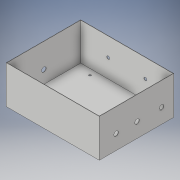
# Autodesk Inventor part: 563-AC-1404-5x4-Enclosure
Saved by Autodesk Inventor 2018 (Build 220112000, 112)
## iProperties
Created: 2018-04-30
Part Number: 563-AC-1404-5x4-Enclosure
Material: Generic
Document SubType Name: Modeling
Designer: bbramman
Density: 1 g/cm^3
Appearance: Default
Author: bbramman
Autodesk Inventor part; units mm, degrees
ref_plane "YZ Plane" through (0, 0, 0) normal (1, 0, 0) x (0, 1, 0)
ref_plane "XZ Plane" through (0, 0, 0) normal (0, 1, 0) x (-1, 0, 0)
ref_plane "XY Plane" through (0, 0, 0) normal (0, 0, 1) x (1, 0, 0)
sketch "Sketch1" plane through (0, 0, 0) normal (0, 1, 0) x (-1, 0, 0)
  line L0 (-63.5, 50.8) -> (63.5, 50.8)
  line L1 (63.5, 50.8) -> (63.5, -50.8)
  line L2 (63.5, -50.8) -> (-63.5, -50.8)
  line L3 (-63.5, -50.8) -> (-63.5, 50.8)
  line L4 (-63.5, 50.8) -> (63.5, -50.8) construction
  line L5 (63.5, 50.8) -> (-63.5, -50.8) construction
  point P0 (0, 0)
  dimension "d0" = 127
  dimension "d1" = 101.6
  constraints: 12 end point, 2 midpoint, 2 parallel, 1 horizontal, 1 perpendicular
  measures "d0" distance of L1.end L2.end
  measures "d1" distance of L0.end L1.end
extrude "Extrusion1" add sketch "Sketch1" along normal blind 1.016
sketch "Sketch2" plane through (0, 1.016, 0) normal (0, 1, 0) x (1, 0, 0)
  line L0 (63.5, 50.8) -> (-63.5, 50.8) projected
  line L1 (63.5, -50.8) -> (-63.5, -50.8)
  line L2 (-63.5, -50.8) -> (-63.5, 50.8)
  line L3 (-63.5, 50.8) -> (63.5, 50.8)
  line L4 (63.5, 50.8) -> (63.5, -50.8)
  line L5 (63.5, -50.8) -> (-63.5, 50.8) construction
  line L6 (-63.5, -50.8) -> (63.5, 50.8) construction
  line L7 (62.992, -50.292) -> (-62.992, -50.292)
  line L8 (-62.992, -50.292) -> (-62.992, 50.292)
  line L9 (-62.992, 50.292) -> (62.992, 50.292)
  line L10 (62.992, 50.292) -> (62.992, -50.292)
  line L11 (62.992, -50.292) -> (-62.992, 50.292) construction
  line L12 (-62.992, -50.292) -> (62.992, 50.292) construction
  point P0 (0, 0)
  dimension "d4" = 125.984
  dimension "d5" = 100.584
  constraints: 24 end point, 4 midpoint, 4 parallel, 2 horizontal, 2 perpendicular
  measures "d4" distance of L8.end L9.end
  measures "d5" distance of L7.end L8.end
extrude "Extrusion2" add sketch "Sketch2" along normal blind 50.8
sketch "Sketch3" plane through (-62.992, 1.016, -50.292) normal (0, 0, 1) x (1, 0, 0)
  line L0 (0, 0) -> (0, 50.8) projected
  circle A0 centre (37.592, 25.4) radius 2.0828
  circle A1 centre (88.392, 25.4) radius 2.0828
  point P0 (62.992, -1.016)
  dimension "d10" = 4.1656
  dimension "d12" = 4.1656
  constraints: 2 centre point
  measures "d10" diameter of A0
  measures "d12" diameter of A1
extrude "Extrusion3" cut sketch "Sketch3" against normal through all
sketch "Sketch4" plane through (-62.992, 1.016, 50.292) normal (1, 0, 0) x (0, 0, -1)
  line L0 (0, 0) -> (0, 50.8) projected
  line L1 (0, 17.581) -> (50.292, 17.581)
  circle A0 centre (50.292, 17.581) radius 3.175
  point P0 (50.292, -1.016)
  dimension "d15" = 6.35
  constraints: 2 end point, 1 centre point, 1 coincident, 1 horizontal, 1 point on line
  measures "d15" diameter of A0
extrude "Extrusion4" cut sketch "Sketch4" against normal through all
sketch "Sketch5" plane through (62.992, 1.016, -50.292) normal (-1, 0, 0) x (0, 0, 1)
  line L0 (0, 0) -> (0, 50.8) projected
  line L1 (0, 19.05) -> (0.2921, 19.05)
  line L2 (0, 19.05) -> (0.2921, 19.05) construction
  line L3 (0.2921, 19.05) -> (16.1671, 19.05)
  line L4 (16.1671, 19.05) -> (49.5173, 19.05)
  line L5 (49.5173, 19.05) -> (20.9423, 19.05)
  line L6 (20.9423, 19.05) -> (49.5173, 19.05)
  line L7 (49.5173, 19.05) -> (78.0923, 19.05)
  circle A0 centre (78.0923, 19.05) radius 3.175
  circle A1 centre (49.5173, 19.05) radius 3.175
  circle A2 centre (16.1671, 19.05) radius 3.175
  point P0 (50.292, -1.016)
  dimension "d18" = 0.2921
  dimension "d19" = 0
  dimension "d20" = 15.875
  dimension "d21" = 33.3502
  dimension "d22" = 180
  dimension "d23" = 28.575
  dimension "d24" = 0
  dimension "d25" = 28.575
  dimension "d26" = 6.35
  dimension "d27" = 6.35
  dimension "d28" = 6.35
  constraints: 14 end point, 4 collinear, 3 centre point, 3 coincident, 3 horizontal, 1 perpendicular, 1 point on line
  measures "d18" distance of L1.start L1.end
  measures "d19" distance between parallel lines of L1 L2
  measures "d20" distance of L2.end L3.end
  measures "d21" distance of L3.end L4.end
  measures "d22" angle of L4 L3
  measures "d23" distance of L4.end L5.end
  measures "d24" distance between parallel lines of L5 L4
  measures "d25" distance of L4.end L7.end
  measures "d26" diameter of A0
  measures "d27" diameter of A1
  measures "d28" diameter of A2
extrude "Extrusion5" cut sketch "Sketch5" against normal through all
sketch "Sketch6" plane through (0, 1.016, 0) normal (0, 1, 0) x (1, 0, 0)
  line L0 (-50, 50) -> (50, -50) construction
  line L1 (50, 50) -> (-50, -50) construction
  circle A0 centre (43.65, 42.38) radius 1.4224
  circle A1 centre (43.65, -42.38) radius 1.4224
  circle A2 centre (-42.38, -42.38) radius 1.4224
  circle A3 centre (-42.38, 42.38) radius 1.4224
  point P0 (0, 0)
  dimension "d31" = 100
  dimension "d32" = 100
  dimension "d38" = 2.8448
  dimension "d39" = 2.8448
  dimension "d40" = 2.8448
  dimension "d41" = 2.8448
  constraints: 4 centre point, 4 end point, 2 midpoint, 1 point on line
  measures "d31" distance of L0.end L1.end
  measures "d32" distance of L1.start L0.end
  measures "d38" diameter of A0
  measures "d39" diameter of A1
  measures "d40" diameter of A2
  measures "d41" diameter of A3
extrude "Extrusion6" cut sketch "Sketch6" against normal through all
body "Solid1"
